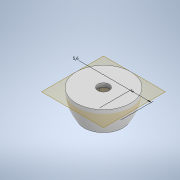
# Autodesk Inventor part: foot
Saved by Autodesk Inventor 2020 (Build 240168000, 168)
## iProperties
Created: 2020-06-05
Part Number: foot
Material: Generic
Document SubType Name: Modeling
Designer: suhren
Density: 1 g/cm^3
Appearance: Default
Author: suhren
Autodesk Inventor part; units mm, degrees
ref_plane "YZ Plane" through (0, 0, 0) normal (1, 0, 0) x (0, 1, 0)
ref_plane "XZ Plane" through (0, 0, 0) normal (0, 1, 0) x (-1, 0, 0)
ref_plane "XY Plane" through (0, 0, 0) normal (0, 0, 1) x (1, 0, 0)
sketch "Sketch1" plane through (0, 0, 0) normal (0, 0, 1) x (1, 0, 0)
  arc A0 (-7.25, 0) -> (-5, -7) centre (4.7639, 0) ccw
  line L0 (-7.25, 0) -> (0, 0)
  line L1 (0, 0) -> (0, -7)
  line L2 (-5, -7) -> (0, -7)
  dimension "d2" = 14.5
  dimension "d3" = 10
  dimension "d4" = 7
  constraints: 7 end point, 2 horizontal, 2 point on circle, 1 centre point, 1 line through centre, 1 vertical
  measures "d2" diameter of L0.start L1
  measures "d3" diameter of L2.start L1
  measures "d4" vertical distance of L0.start L2.start
revolve "Revolution1" add sketch "Sketch1" angle 360 about axis through (0, 0, 0) along (0, -1, 0)
sketch "Sketch2" plane through (0, -7, 0) normal (0, -1, 0) x (1, 0, 0)
  line L0 (-2.8, 1.6166) -> (0, 3.2332)
  line L1 (0, 3.2332) -> (2.8, 1.6166)
  line L2 (2.8, 1.6166) -> (2.8, -1.6166)
  line L3 (2.8, -1.6166) -> (0, -3.2332)
  line L4 (0, -3.2332) -> (-2.8, -1.6166)
  line L5 (-2.8, -1.6166) -> (-2.8, 1.6166)
  point P0 (0, 0)
  point P1 (0, 0)
  dimension "d6" = 5.6
  constraints: 12 end point, 1 coincident, 1 vertical, 13 other
  measures "d6" distance between parallel lines of L5 L2
ref_plane "Work Plane1" through (0, -1, 0) normal (0, 1, 0) x (1, 0, 0)
extrude "Extrusion1" cut sketch "Sketch2" against normal up to surface (6 mm away)
hole "Hole1" at (0, -7, 0) direction (0, 1, 0) diameter 3 end through all
fillet "Fillet1" radius 0.5 7 edges at (-1.4, -7, 2.4249) (-2.8, -7, 0) (-1.4, -7, -2.4249) (1.4, -7, -2.4249) (2.8, -7, 0) (1.4, -7, 2.4249) (5, -7, 0)
body "Solid1"
